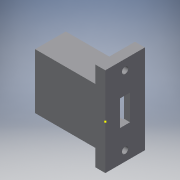
# Autodesk Inventor part: USB_housing
Saved by Autodesk Inventor 2018 (Build 220112000, 112)
## iProperties
Created: 2018-05-29
Part Number: USB_housing
Material: Generic
Document SubType Name: Sheet Metal
Designer: David
Density: 1 g/cm^3
Appearance: Default
Sheet Metal Rule: Default
Author: David
Autodesk Inventor part; units mm, degrees
ref_plane "YZ Plane" through (0, 0, 0) normal (1, 0, 0) x (0, 1, 0)
ref_plane "XZ Plane" through (0, 0, 0) normal (0, 1, 0) x (-1, 0, 0)
ref_plane "XY Plane" through (0, 0, 0) normal (0, 0, 1) x (1, 0, 0)
sketch "Sketch1" plane through (0, 0, 0) normal (1, 0, 0) x (0, 1, 0)
  line L0 (-2.5, -6.5) -> (2.5, -6.5)
  line L1 (2.5, -6.5) -> (2.5, 6.5)
  line L2 (2.5, 6.5) -> (-2.5, 6.5)
  line L3 (-2.5, 6.5) -> (-2.5, -6.5)
  line L4 (-2.5, -6.5) -> (2.5, 6.5) construction
  line L5 (2.5, -6.5) -> (-2.5, 6.5) construction
  line L6 (-10, -22.5) -> (10, -22.5)
  line L7 (10, -22.5) -> (10, 22.5)
  line L8 (10, 22.5) -> (-10, 22.5)
  line L9 (-10, 22.5) -> (-10, -22.5)
  line L10 (-10, -22.5) -> (10, 22.5) construction
  line L11 (10, -22.5) -> (-10, 22.5) construction
  circle A0 centre (2.5, 17.5) radius 1.6
  circle A1 centre (0, -17.5) radius 1.6
  point P0 (0, 0)
  dimension "d0" = 5
  dimension "d1" = 13
  dimension "d2" = 20
  dimension "d3" = 45
  dimension "d17" = 5
  dimension "d18" = 3.2
  dimension "d19" = 3.2
  dimension "d20" = 5
  constraints: 24 end point, 4 midpoint, 4 parallel, 2 centre point, 2 horizontal, 2 perpendicular
  measures "d0" distance of L2.end L1.end
  measures "d1" distance of L1.end L0.end
  measures "d2" distance of L8.end L7.end
  measures "d3" distance of L7.end L6.end
  measures "d17" distance from line of L8 A0.centre
  measures "d18" diameter of A0
  measures "d19" diameter of A1
  measures "d20" distance from line of L6 A1.centre
extrude "Extrusion1" add sketch "Sketch1" against normal blind 5 contours L9 L8 L7 L6 | A0 | A1
sketch "Sketch2" plane through (-5, 0, 0) normal (-1, 0, 0) x (0, 0, 1)
  line L0 (10, -5.5) -> (-10, -5.5)
  line L1 (-10, -5.5) -> (-10, 5.5)
  line L2 (-10, 5.5) -> (10, 5.5)
  line L3 (10, 5.5) -> (10, -5.5)
  line L4 (10, -5.5) -> (-10, 5.5) construction
  line L5 (-10, -5.5) -> (10, 5.5) construction
  line L6 (22.5, 10) -> (-22.5, 10) projected
  line L7 (-14, -10) -> (-14, 5.5)
  line L8 (14, 5.5) -> (14, -10)
  line L9 (12.0522, -8.6087) -> (-14, 10) construction
  line L10 (-12.0522, -8.6087) -> (14, 10) construction
  line L11 (-14, -10) -> (14, -10)
  line L12 (-14, 5.5) -> (14, 5.5)
  point P0 (0, 0)
  dimension "d6" = 20
  dimension "d7" = 11
  dimension "d27" = 4.5
  dimension "d32" = 14
  dimension "d33" = 14
  constraints: 24 end point, 3 parallel, 3 perpendicular, 3 point on line, 2 midpoint, 1 horizontal
  measures "d6" distance of L1.end L2.end
  measures "d7" distance of L0.end L1.end
  measures "d27" distance between parallel lines of L0 L11
  measures "d32" distance from line of point (0, 0) L7
  measures "d33" distance from line of L8 point (0, 0)
extrude "Extrusion2" add sketch "Sketch2" along normal blind 27 contours L3 L12 L8 L11 L7 L1 L0
sketch "Sketch3" plane through (0, -10, -22.5) normal (0, -1, 0) x (1, 0, 0)
  point P0 (0, 22.5)
sketch "Sketch4" plane through (-32, 0, 0) normal (-1, 0, 0) x (0, 0, 1)
  line L0 (6.5, -5.5) -> (-6.5, -5.5)
  line L1 (-6.5, -5.5) -> (-6.5, 5.5)
  line L2 (-6.5, 5.5) -> (6.5, 5.5)
  line L3 (6.5, 5.5) -> (6.5, -5.5)
  line L4 (6.5, -5.5) -> (-6.5, 5.5) construction
  line L5 (-6.5, -5.5) -> (6.5, 5.5) construction
  line L6 (12.0522, -8.6087) -> (-14, 10) construction
  line L7 (-12.5, -10) -> (12.5, 10) construction
  line L8 (14, -10) -> (14, 5.5) projected
  line L9 (-14, -10) -> (14, -10)
  line L10 (14, -10) -> (14, 5.5)
  line L11 (14, 5.5) -> (-14, 5.5)
  line L12 (-14, 5.5) -> (-14, -10)
  point P0 (0, 0)
  point P1 (14, 10)
  dimension "d11" = 13
  dimension "d12" = 11
  constraints: 25 end point, 4 parallel, 3 midpoint, 2 horizontal, 2 perpendicular, 1 point on line
  measures "d11" distance of L1.end L2.end
  measures "d12" distance of L0.end L1.end
sketch "Sketch6" plane through (0, 0, 0) normal (1, 0, 0) x (0, 0, -1)
  circle A0 centre (17.5, 0) radius 1.6
  circle A1 centre (-17.5, 0) radius 1.6
  line L0 (22.5, -10) -> (22.5, 10) projected
  line L1 (-22.5, 10) -> (-22.5, -10) projected
  line L2 (22.5, -10) -> (14, -10) projected
  point P0 (0, 0)
  dimension "d21" = 3.2
  dimension "d22" = 3.2
  dimension "d23" = 5
  dimension "d24" = 5
  dimension "d41" = 10
  constraints: 2 centre point
  measures "d21" diameter of A0
  measures "d22" diameter of A1
  measures "d23" distance from line of L0 A0.centre
  measures "d24" distance from line of L1 A1.centre
  measures "d41" distance from line of L2 A0.centre
extrude "Extrusion5" cut sketch "Sketch6" against normal blind 5
extrude "Extrusion8" add sketch "Sketch4" along normal blind 3.5 contours L3 L11 L8 L9 L12 L1 L0
sketch "Sketch8" plane through (-5, 0, 0) normal (-1, 0, 0) x (0, 0, 1)
  line L0 (-10, 5.5) -> (-10, -5.5) projected
  line L1 (-10, -5.5) -> (10, -5.5)
  line L2 (10, -5.5) -> (10, 6.5)
  line L3 (10, 6.5) -> (-10, 6.5)
  line L4 (-10, 6.5) -> (-10, -5.5)
  point P0 (0, 0)
  dimension "d36" = 12
  constraints: 8 end point, 2 parallel, 1 horizontal, 1 perpendicular
  measures "d36" distance of L1.end L2.end
extrude "Extrusion10" cut sketch "Sketch8" against normal blind 2
equation "\"BendRadius\" = Thickness"
equation "\"BendReliefWidth\" = Thickness"
equation "\"BendReliefDepth\" = 0.5 * Thickness"
equation "\"CornerReliefSize\" = 4 * Thickness"
equation "\"MinimumRemnant\" = 2 * Thickness"
equation "\"TransitionRadius\" = BendRadius"
equation "\"JacobiRadiusSize\" = Thickness"
equation "\"GapSize\" = Thickness"
equation "\"Thickness\" = 0.5"
body "Solid1"
